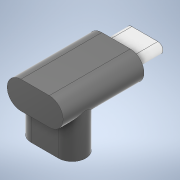
# Autodesk Inventor part: usb_connect
Saved by Autodesk Inventor 2020 (Build 240168000, 168)
## iProperties
Created: 2023-09-20
Part Number: usb_connect
Material: 일반
Document SubType Name: Modeling
Designer: ac837
Density: 1 g/cm^3
Appearance: 기본값
Author: ac837
Autodesk Inventor part; units mm, degrees
ref_plane "YZ Plane" through (0, 0, 0) normal (1, 0, 0) x (0, 1, 0)
ref_plane "XZ Plane" through (0, 0, 0) normal (0, 1, 0) x (-1, 0, 0)
ref_plane "XY Plane" through (0, 0, 0) normal (0, 0, 1) x (1, 0, 0)
sketch "스케치1" plane through (0, 0, 0) normal (0, 0, 1) x (1, 0, 0)
  line L0 (0, 0) -> (8.4, 0)
  line L1 (8.4, 0) -> (8.4, 2.38)
  line L2 (8.4, 2.38) -> (0, 2.38)
  line L3 (0, 2.38) -> (0, 0)
  dimension "d0" = 8.4
  dimension "d1" = 2.38
  constraints: 8 end point, 2 parallel, 1 horizontal, 1 perpendicular
  measures "d0" distance of L2.end L1.end
  measures "d1" distance of L1.end L0.end
extrude "돌출1" add sketch "스케치1" along normal blind 6.7
fillet "모깎기1" radius 1.19 4 edges at (8.4, 2.38, 3.35) (8.4, 0, 3.35) (0, 2.38, 3.35) (0, 0, 3.35)
sketch "스케치2" plane through (0, 0, 0) normal (0, 0, -1) x (-1, 0, 0)
  arc A0 (-7.21, 2.38) -> (-7.21, 0) centre (-7.21, 1.19) ccw projected
  arc A1 (-1.19, 0) -> (-1.19, 2.38) centre (-1.19, 1.19) ccw projected
  line L0 (-7.21, 2.38) -> (-1.19, 2.38) projected
  arc A2 (-7.21, 2.38) -> (-7.21, 0) centre (-7.21, 1.19) ccw projected
  line L1 (-1.19, 0) -> (-7.21, 0) projected
  arc A3 (-1.19, 0.3) -> (-1.19, 2.08) centre (-1.19, 1.19) ccw
  line L2 (-1.19, 0.3) -> (-7.21, 0.3)
  arc A4 (-7.21, 2.08) -> (-7.21, 0.3) centre (-7.21, 1.19) ccw
  line L3 (-7.21, 2.08) -> (-1.19, 2.08)
  point P0 (0, 0)
  dimension "d5" = 0.3
  constraints: 4 end point, 4 point on circle, 2 centre point, 3 other
  measures "d5" distance between parallel lines of L0 L3
extrude "돌출2" cut sketch "스케치2" against normal blind 6 contours L2 A4 L3 A3
sketch "스케치3" plane through (0, 0, 6.7) normal (0, 0, 1) x (1, 0, 0)
  line L0 (7.21, 2.38) -> (1.19, 2.38) projected
  line L1 (4.2, 2.38) -> (4.2, 0)
  line L2 (1.19, 0) -> (7.21, 0) projected
  line L3 (4.2, 1.19) -> (0, 1.19)
  arc A0 (1.19, 2.38) -> (1.19, 0) centre (1.19, 1.19) ccw projected
  line L4 (4.2, 1.19) -> (8.4, 1.19)
  arc A1 (7.21, 0) -> (7.21, 2.38) centre (7.21, 1.19) ccw projected
  line L5 (-2.3, -2.01) -> (10.7, -2.01)
  line L6 (10.7, -2.01) -> (10.7, 4.39)
  line L7 (10.7, 4.39) -> (-2.3, 4.39)
  line L8 (-2.3, 4.39) -> (-2.3, -2.01)
  line L9 (-2.3, -2.01) -> (10.7, 4.39) construction
  line L10 (10.7, -2.01) -> (-2.3, 4.39) construction
  line L11 (-2.3, -2.01) -> (10.7, -2.01) construction
  point P0 (0, 0)
  dimension "d8" = 13
  dimension "d9" = 0
  dimension "d10" = 6.4
  constraints: 20 end point, 5 midpoint, 3 perpendicular, 2 parallel, 2 point on circle, 1 collinear, 1 horizontal, 1 point on line
  measures "d8" distance of L5.start L5.end
  measures "d9" distance between parallel lines of L5 L11
  measures "d10" distance of L6.end L5.end
extrude "돌출3" add sketch "스케치3" along normal blind 18.8 contours A1 L4 L1 L0 | L1 L3 A0 L0 | A1 L2 L1 L4 | L1 L2 A0 L3 | L8 L7 L6 L5
fillet "모깎기2" radius 3.2 4 edges at (10.7, 4.39, 16.1) (10.7, -2.01, 16.1) (-2.3, 4.39, 16.1) (-2.3, -2.01, 16.1)
sketch "스케치4" plane through (0.9, -2.01, 6.7) normal (0, -1, 0) x (1, 0, 0)
  line L0 (0.29, 0) -> (6.31, 0) projected
  line L1 (3.3, 0) -> (3.3, 13.4)
  line L2 (3.3, 0) -> (16.7, 0) construction
  line L3 (9.65, 16.55) -> (-3.05, 16.55)
  line L4 (-3.05, 16.55) -> (-3.05, 10.25)
  line L5 (-3.05, 10.25) -> (9.65, 10.25)
  line L6 (9.65, 10.25) -> (9.65, 16.55)
  line L7 (9.65, 16.55) -> (-3.05, 10.25) construction
  line L8 (-3.05, 16.55) -> (9.65, 10.25) construction
  line L9 (9.65, 16.55) -> (22.35, 16.55) construction
  point P0 (-0.9, -6.7)
  dimension "d14" = 13.4
  dimension "d15" = 90
  dimension "d16" = 12.7
  dimension "d17" = 180
  dimension "d18" = 6.3
  constraints: 18 end point, 3 horizontal, 3 midpoint, 2 equal length, 2 parallel, 1 perpendicular, 1 vertical
  measures "d14" distance of L1.start L1.end
  measures "d15" angle of L2 L1
  measures "d16" distance of L3.start L3.end
  measures "d17" angle of L3 L9
  measures "d18" distance of L4.end L3.end
extrude "돌출4" add sketch "스케치4" along normal blind 7.4 and the other way blind 3
fillet "모깎기3" radius 3.15 4 edges at (10.55, -4.5943, 16.95) (10.55, -4.5943, 23.25) (-2.15, -4.5943, 16.95) (-2.15, -4.5943, 23.25)
sketch "스케치5" plane through (0.9, -9.41, 6.7) normal (0, -1, 0) x (1, 0, 0)
  arc A0 (0.1, 16.55) -> (0.1, 10.25) centre (0.1, 13.4) ccw projected
  line L0 (0.1, 10.25) -> (6.5, 10.25) projected
  arc A1 (6.5, 10.25) -> (6.5, 16.55) centre (6.5, 13.4) ccw projected
  line L1 (6.5, 16.55) -> (0.1, 16.55) projected
  line L2 (6.5, 11.85) -> (0.1, 11.85)
  arc A2 (0.1, 14.95) -> (0.1, 11.85) centre (0.1, 13.4) ccw
  line L3 (0.1, 14.95) -> (6.5, 14.95)
  arc A3 (6.5, 11.85) -> (6.5, 14.95) centre (6.5, 13.4) ccw
  point P0 (-0.9, -6.7)
  dimension "d24" = 1.6
  constraints: 4 end point, 4 point on circle, 2 centre point, 3 other
  measures "d24" distance between parallel lines of L0 L2
extrude "돌출5" cut sketch "스케치5" against normal blind 9.6 contours L2 A2 L3 A3
